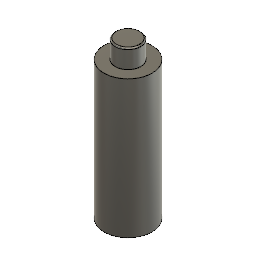
_Sorter Leg.fef3ed54-a3fd-402f-8981-d6e8346332c7 (Autodesk Fusion 360 design; units mm, degrees)
Autodesk Fusion 360 part; units mm, degrees
sketch "Sketch1" plane through (0, 0, 0) normal (0, 1, 0) x (1, 0, 0)
  circle A0 centre (0, 0) radius 7.5
  line L0 (6.4897, 0.2677) -> (3.013, 5.7541)
  line L1 (3.013, 5.7541) -> (-3.4767, 5.4864)
  line L2 (-3.4767, 5.4864) -> (-6.4897, -0.2677)
  line L3 (-6.4897, -0.2677) -> (-3.013, -5.7541)
  line L4 (-3.013, -5.7541) -> (3.4767, -5.4864)
  line L5 (3.4767, -5.4864) -> (6.4897, 0.2677)
  circle A1 centre (0, 0) radius 3.55
  dimension "d1" = 15
  dimension "d2" = 5.625
  dimension "d7" = 7.1
  constraint coincident A0.centre A1.centre
  constraint concentric A0 A1
  measures "d1" diameter of A0
  measures "d2" distance of A0.centre L5
  measures "d7" diameter of A1
extrude "Extrude1" add sketch "Sketch1" along normal blind 42.88 contours A0 | L0 L1 L2 L3 L4 L5 | A1
extrude "Extrude2" cut sketch "Sketch1" along normal blind 5.9 contours L0 L1 L2 L3 L4 L5 | A1
extrude "Extrude3" cut sketch "Sketch1" along normal blind 39 contours A1
sketch "Sketch2" plane through (0, 42.88, 0) normal (0, 1, 0) x (-1, 0, 0)
  circle A0 centre (0, 0) radius 7.5
  circle A1 centre (0, 0) radius 3.98
  dimension "d10" = 7.96
  constraint coincident A0.centre A1.centre
  measures "d10" diameter of A1
extrude "Extrude4" add sketch "Sketch2" along normal blind 5.8 contours A1
fillet "Fillet1" radius 0.4 1 edges at (3.7107, 48.68, -1.4392)
